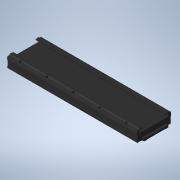
# Autodesk Inventor part: ETH2-17-L5-350-BC-M40B-C6N5L_1
Saved by Autodesk Inventor 2021 (Build 250183000, 183)
## iProperties
Created: 2025-05-01
Part Number: ETH2-17-L5-350-BC-M40B-C6N5L_1
Material: Generic
Catalog Web Link: www.cadenas.de
Description: ETH2_17_1-ETH2
Vendor: TOYO
Document SubType Name: Modeling
Designer: psAdmin
Manufacturer: TOYO
Mass: 3122.58 g
Surface Area: 3378.61 cm^2
Volume: 3122.58 cm^3
Density: 1 g/cm^3
Appearance: PSOLRGB-175-175-175
Category: PARTsolutions
Company: TOYO
Title: ETH2-17-L5-350-BC-M40B-C6N5L
Author: Cadenas PARTsolutions
Comments: ETH2
PSOL_IDENT_0: {$CADENAS_DATA/23d-libs/toyo/eth2_series/eth2_17/parts/eth2_17_body1.prj},242 {VTYP=3D},{NB=ETH2-17-
PSOL_IDENT_1: L5-350-BC-M40B-C6N5L_1},{LINA=ETH2-17-L5-350-BC-M40B-C6N5L},{NN=ETH2_17_1},{DATE=15.08.2024 07:04:56
PSOL_IDENT_2: },{GEOMDATE=05.08.2024 03:26:00},{VERSION=},{LINEID=10},{WBVAR=BSL,STROKE,MP,MB,BRAKE,HS,LS,OML,SD},
PSOL_IDENT_3: {WBNUMERIC=STROKE}  {NB=ETH2-17-L5-350-BC-M40B-C6N5L_1},{LINA=ETH2-17-L5-350-BC-M40B-C6N5L},{KT=DUMM
PSOL_IDENT_4: Y},{CNSORDERNO=ETH2-17-L5-350-BC-M40B-C6N5L},{MODEL=ETH2-17},{BSL=5},{BSL1=5},{STROKE=350},{MP=BC},{
PSOL_IDENT_5: MB=M},{POWEWR=40：400W},{BRAKE=B},{HS=C},{LS=6},{LS1='3','3:1 Pc','4','4:2 Pc','6','6:3 Pc','7','7:4
PSOL_IDENT_6: Pc','8','8:5 Pc','9','9:6 Pc','5','5:No Sensor'},{OML=N5},{SD=L},{L=615},{A=69},{A1=69},{M=4},{N=10}
PSOL_IDENT_7: ,{KG=9.42},{HLS=C6},{LSLIDER=1},{RSLIDRE=0},{MBCODE=M40B}
NB: ETH2-17-L5-350-BC-M40B-C6N5L_1
NN: ETH2_17_1
NT: ETH2
NBSYN: $CNSORDERNO._1
LINA: ETH2-17-L5-350-BC-M40B-C6N5L
CATALOG: TOYO
MODEL: ETH2-17
BSL: 5:5mm
STROKE: 350
MP: BC:Motor Exposed
MB: M:Mitsubishi
POWEWR: 40：400W
BRAKE: B:With brake
HS: C:Motor Side
LS: 6:3 Pc
OML: N5:NPN+5 meter cable
SD: L: Left side of slide
SUPPLIER: TOYO
ARTICLENO: ETH2-17-L5-350-BC-M40B-C6N5L_1
BOMINFO: ETH2-17-L5-350-BC-M40B-C6N5L
CREATOR: CADENAS GmbH
Autodesk Inventor part; units mm, degrees
sketch "__4" plane through (0, 0, 0) normal (1, 0, 0) x (0, 1, 0)
  line L0 (43, 79) -> (41.05, 79)
  arc A0 (41.05, 79) -> (40.75, 78.7) centre (41.05, 78.7) ccw
  line L1 (40.75, 78.7) -> (40.75, 77.8)
  arc A1 (40.75, 77.8) -> (41.05, 77.5) centre (41.05, 77.8) ccw
  line L2 (41.05, 77.5) -> (41.55, 77.5)
  arc A2 (41.85, 77.2) -> (41.55, 77.5) centre (41.55, 77.2) ccw
  line L3 (41.85, 77.2) -> (41.85, 75.1743)
  arc A3 (41.7621, 74.9621) -> (41.85, 75.1743) centre (41.55, 75.1743) ccw
  line L4 (41.7621, 74.9621) -> (40.6879, 73.8879)
  arc A4 (40.4757, 73.8) -> (40.6879, 73.8879) centre (40.4757, 74.1) ccw
  line L5 (40.4757, 73.8) -> (37.5243, 73.8)
  arc A5 (37.3121, 73.8879) -> (37.5243, 73.8) centre (37.5243, 74.1) ccw
  line L6 (37.3121, 73.8879) -> (36.2379, 74.9621)
  arc A6 (36.15, 75.1743) -> (36.2379, 74.9621) centre (36.45, 75.1743) ccw
  line L7 (36.15, 75.1743) -> (36.15, 77.2)
  arc A7 (36.45, 77.5) -> (36.15, 77.2) centre (36.45, 77.2) ccw
  line L8 (36.45, 77.5) -> (36.95, 77.5)
  arc A8 (36.95, 77.5) -> (37.25, 77.8) centre (36.95, 77.8) ccw
  line L9 (37.25, 77.8) -> (37.25, 78.7)
  arc A9 (37.25, 78.7) -> (36.95, 79) centre (36.95, 78.7) ccw
  line L10 (36.95, 79) -> (35, 79)
  arc A10 (35, 79) -> (34, 78) centre (35, 78) ccw
  line L11 (34, 78) -> (34, 75.8)
  arc A11 (33.5, 75.3) -> (34, 75.8) centre (33.5, 75.8) ccw
  line L12 (33.5, 75.3) -> (10.8243, 75.3)
  arc A12 (10.6121, 75.3879) -> (10.8243, 75.3) centre (10.8243, 75.6) ccw
  line L13 (10.6121, 75.3879) -> (10.0879, 75.9121)
  arc A13 (10.0879, 75.9121) -> (9.8757, 76) centre (9.8757, 75.7) ccw
  line L14 (9.8757, 76) -> (0.6243, 76)
  arc A14 (0.6243, 76) -> (0.4121, 75.9121) centre (0.6243, 75.7) ccw
  line L15 (0.4121, 75.9121) -> (0, 75.5)
  line L16 (0, 75.5) -> (0, 39.5)
  line L17 (0, 39.5) -> (0.9121, 38.5879)
  arc A15 (1, 38.3757) -> (0.9121, 38.5879) centre (0.7, 38.3757) ccw
  line L18 (1, 38.3757) -> (1, -38.3757)
  arc A16 (0.9121, -38.5879) -> (1, -38.3757) centre (0.7, -38.3757) ccw
  line L19 (0.9121, -38.5879) -> (0, -39.5)
  line L20 (0, -39.5) -> (0, -75.5)
  line L21 (0, -75.5) -> (0.5, -76)
  line L22 (0.5, -76) -> (10, -76)
  line L23 (10, -76) -> (10.6121, -75.3879)
  arc A17 (10.8243, -75.3) -> (10.6121, -75.3879) centre (10.8243, -75.6) ccw
  line L24 (10.8243, -75.3) -> (26.1757, -75.3)
  arc A18 (26.3879, -75.3879) -> (26.1757, -75.3) centre (26.1757, -75.6) ccw
  line L25 (26.3879, -75.3879) -> (28, -77)
  line L26 (28, -77) -> (45, -77)
  line L27 (45, -77) -> (46.9121, -75.0879)
  arc A19 (46.9121, -75.0879) -> (47, -74.8757) centre (46.7, -74.8757) ccw
  line L28 (47, -74.8757) -> (47, -69.3743)
  arc A20 (47.0879, -69.1621) -> (47, -69.3743) centre (47.3, -69.3743) ccw
  line L29 (47.0879, -69.1621) -> (51.4121, -64.8379)
  arc A21 (51.4121, -64.8379) -> (51.5, -64.6257) centre (51.2, -64.6257) ccw
  line L30 (51.5, -64.6257) -> (51.5, -61.9243)
  arc A22 (51.5, -61.9243) -> (51.4121, -61.7121) centre (51.2, -61.9243) ccw
  line L31 (51.4121, -61.7121) -> (51.2879, -61.5879)
  arc A23 (51.2, -61.3757) -> (51.2879, -61.5879) centre (51.5, -61.3757) ccw
  line L32 (51.2, -61.3757) -> (51.2, -56.8)
  arc A24 (51.2, -56.8) -> (50.9, -56.5) centre (50.9, -56.8) ccw
  line L33 (50.9, -56.5) -> (50.259, -56.5)
  arc A25 (49.141, -56.5) -> (50.259, -56.5) centre (49.7, -56) ccw
  line L34 (49.141, -56.5) -> (48.5, -56.5)
  arc A26 (48.2, -56.2) -> (48.5, -56.5) centre (48.5, -56.2) ccw
  line L35 (48.2, -56.2) -> (48.2, -52.8)
  arc A27 (48.5, -52.5) -> (48.2, -52.8) centre (48.5, -52.8) ccw
  line L36 (48.5, -52.5) -> (49.141, -52.5)
  arc A28 (50.259, -52.5) -> (49.141, -52.5) centre (49.7, -53) ccw
  line L37 (50.259, -52.5) -> (50.9, -52.5)
  arc A29 (50.9, -52.5) -> (51.2, -52.2) centre (50.9, -52.2) ccw
  line L38 (51.2, -52.2) -> (51.2, -51.5)
  arc A30 (51.2, -51.5) -> (50.7, -51) centre (50.7, -51.5) ccw
  line L39 (50.7, -51) -> (47, -51)
  arc A31 (47, -51) -> (45.5, -52.5) centre (47, -52.5) ccw
  line L40 (45.5, -52.5) -> (45.5, -61.3762)
  arc A32 (45.5, -61.3762) -> (45.673, -61.648) centre (45.8, -61.3762) ccw
  line L41 (45.673, -61.648) -> (45.708, -61.664)
  arc A33 (45.708, -61.664) -> (46.084, -61.559) centre (45.8347, -61.3921) ccw
  arc A34 (46.269, -63.673) -> (46.084, -61.559) centre (47.4997, -62.5002) ccw
  arc A35 (46.269, -63.673) -> (45.8797, -63.6342) centre (46.0518, -63.8799) ccw
  line L42 (45.8797, -63.6342) -> (43.4739, -65.3191)
  arc A36 (42.9002, -65.5) -> (43.4739, -65.3191) centre (42.9002, -64.5) ccw
  line L43 (42.9002, -65.5) -> (32.748, -65.5)
  line L44 (32.748, -65.5) -> (32.748, 65.5)
  line L45 (32.748, 65.5) -> (42.9002, 65.5)
  arc A37 (43.4739, 65.3191) -> (42.9002, 65.5) centre (42.9002, 64.5) ccw
  line L46 (43.4739, 65.3191) -> (45.8797, 63.6342)
  arc A38 (45.8797, 63.6342) -> (46.269, 63.673) centre (46.0518, 63.8799) ccw
  arc A39 (46.084, 61.559) -> (46.269, 63.673) centre (47.4997, 62.5002) ccw
  arc A40 (46.084, 61.559) -> (45.708, 61.664) centre (45.8347, 61.3921) ccw
  line L47 (45.708, 61.664) -> (45.673, 61.648)
  arc A41 (45.673, 61.648) -> (45.5, 61.3762) centre (45.8, 61.3762) ccw
  line L48 (45.5, 61.3762) -> (45.5, 52.5)
  arc A42 (45.5, 52.5) -> (47, 51) centre (47, 52.5) ccw
  line L49 (47, 51) -> (50.7, 51)
  arc A43 (50.7, 51) -> (51.2, 51.5) centre (50.7, 51.5) ccw
  line L50 (51.2, 51.5) -> (51.2, 52.2)
  arc A44 (51.2, 52.2) -> (50.9, 52.5) centre (50.9, 52.2) ccw
  line L51 (50.9, 52.5) -> (50.259, 52.5)
  arc A45 (49.141, 52.5) -> (50.259, 52.5) centre (49.7, 53) ccw
  line L52 (49.141, 52.5) -> (48.5, 52.5)
  arc A46 (48.2, 52.8) -> (48.5, 52.5) centre (48.5, 52.8) ccw
  line L53 (48.2, 52.8) -> (48.2, 56.2)
  arc A47 (48.5, 56.5) -> (48.2, 56.2) centre (48.5, 56.2) ccw
  line L54 (48.5, 56.5) -> (49.141, 56.5)
  arc A48 (50.259, 56.5) -> (49.141, 56.5) centre (49.7, 56) ccw
  line L55 (50.259, 56.5) -> (50.9, 56.5)
  arc A49 (50.9, 56.5) -> (51.2, 56.8) centre (50.9, 56.8) ccw
  line L56 (51.2, 56.8) -> (51.2, 61.3757)
  arc A50 (51.2879, 61.5879) -> (51.2, 61.3757) centre (51.5, 61.3757) ccw
  line L57 (51.2879, 61.5879) -> (51.4121, 61.7121)
  arc A51 (51.4121, 61.7121) -> (51.5, 61.9243) centre (51.2, 61.9243) ccw
  line L58 (51.5, 61.9243) -> (51.5, 64.6257)
  arc A52 (51.5, 64.6257) -> (51.4121, 64.8379) centre (51.2, 64.6257) ccw
  line L59 (51.4121, 64.8379) -> (47.0879, 69.1621)
  arc A53 (47, 69.3743) -> (47.0879, 69.1621) centre (47.3, 69.3743) ccw
  line L60 (47, 69.3743) -> (47, 74.8757)
  arc A54 (47, 74.8757) -> (46.9121, 75.0879) centre (46.7, 74.8757) ccw
  line L61 (46.9121, 75.0879) -> (46.0879, 75.9121)
  arc A55 (46.0879, 75.9121) -> (45.8757, 76) centre (45.8757, 75.7) ccw
  line L62 (45.8757, 76) -> (44.5, 76)
  arc A56 (44, 76.5) -> (44.5, 76) centre (44.5, 76.5) ccw
  line L63 (44, 76.5) -> (44, 78)
  arc A57 (44, 78) -> (43, 79) centre (43, 78) ccw
  constraints: 128 end point, 116 point on circle, 58 centre point
extrude "Extrusion1" add sketch "__4" along normal blind 596
sketch "__1" plane through (0, 0, 0) normal (0, 1, 0) x (-1, 0, 0)
  line L0 (-586, 90) -> (-606, 90)
  line L1 (-606, 90) -> (-606, -90)
  line L2 (-606, -90) -> (-586, -90)
  line L3 (-586, -90) -> (-586, -60.5)
  arc A0 (-586, -60.5) -> (-592, -54.5) centre (-592, -60.5) ccw
  line L4 (-592, -54.5) -> (-596, -54.5)
  line L5 (-596, -54.5) -> (-596, 54.5)
  line L6 (-596, 54.5) -> (-592, 54.5)
  arc A1 (-592, 54.5) -> (-586, 60.5) centre (-592, 60.5) ccw
  line L7 (-586, 60.5) -> (-586, 90)
  constraints: 16 end point, 4 point on circle, 2 centre point
extrude "Extrusion2" cut sketch "__1" along normal blind 51.5
sketch "__3" plane through (596, 0, 0) normal (1, 0, 0) x (0, 0, -1)
  line L0 (-90, 70) -> (-90, 0)
  line L1 (-90, 0) -> (-60.5, 0)
  line L2 (-60.5, 0) -> (-60.5, 12.8)
  line L3 (-60.5, 12.8) -> (-58.4243, 12.8)
  arc A0 (-58.2121, 12.7121) -> (-58.4243, 12.8) centre (-58.4243, 12.5) ccw
  line L4 (-58.2121, 12.7121) -> (-56.0879, 10.5879)
  arc A1 (-56.0879, 10.5879) -> (-55.8757, 10.5) centre (-55.8757, 10.8) ccw
  line L5 (-55.8757, 10.5) -> (-55.6243, 10.5)
  arc A2 (-55.6243, 10.5) -> (-55.4121, 10.5879) centre (-55.6243, 10.8) ccw
  line L6 (-55.4121, 10.5879) -> (-55, 11)
  line L7 (-55, 11) -> (-39, 11)
  line L8 (-39, 11) -> (-37.5879, 9.5879)
  arc A3 (-37.5879, 9.5879) -> (-37.3757, 9.5) centre (-37.3757, 9.8) ccw
  line L9 (-37.3757, 9.5) -> (-30.1243, 9.5)
  arc A4 (-30.1243, 9.5) -> (-29.9121, 9.5879) centre (-30.1243, 9.8) ccw
  line L10 (-29.9121, 9.5879) -> (-29.5, 10)
  line L11 (-29.5, 10) -> (-17.5, 10)
  line L12 (-17.5, 10) -> (-17.0879, 9.5879)
  arc A5 (-17.0879, 9.5879) -> (-16.8757, 9.5) centre (-16.8757, 9.8) ccw
  line L13 (-16.8757, 9.5) -> (16.8757, 9.5)
  arc A6 (16.8757, 9.5) -> (17.0879, 9.5879) centre (16.8757, 9.8) ccw
  line L14 (17.0879, 9.5879) -> (17.5, 10)
  line L15 (17.5, 10) -> (27.634, 10)
  arc A7 (27.634, 10) -> (29, 11.366) centre (28.5001, 10.4999) ccw
  line L16 (29, 11.366) -> (29, 12)
  line L17 (29, 12) -> (30.8757, 12)
  arc A8 (31.0879, 11.9121) -> (30.8757, 12) centre (30.8757, 11.7) ccw
  line L18 (31.0879, 11.9121) -> (32.5121, 10.4879)
  arc A9 (32.5121, 10.4879) -> (32.7243, 10.4) centre (32.7243, 10.7) ccw
  line L19 (32.7243, 10.4) -> (38.2757, 10.4)
  arc A10 (38.2757, 10.4) -> (38.4879, 10.4879) centre (38.2757, 10.7) ccw
  line L20 (38.4879, 10.4879) -> (39, 11)
  line L21 (39, 11) -> (53.134, 11)
  arc A11 (53.134, 11) -> (54.5, 10.634) centre (54, 11.5) ccw
  arc A12 (54.5, 10.634) -> (54.866, 11) centre (54, 11.5) ccw
  line L22 (54.866, 11) -> (60.5, 11)
  line L23 (60.5, 11) -> (60.5, 0)
  line L24 (60.5, 0) -> (90, 0)
  line L25 (90, 0) -> (90, 70)
  line L26 (90, 70) -> (-90, 70)
  constraints: 54 end point, 26 point on circle, 13 centre point
extrude "Extrusion3" cut sketch "__3" against normal blind 10
sketch "__5" plane through (0, 0, 70) normal (0, 0, 1) x (1, 0, 0)
  line L0 (51, 51.5) -> (51, 0)
  line L1 (51, 0) -> (48, 0)
  line L2 (48, 0) -> (48.5415, 0.5415)
  line L3 (48.5415, 0.5415) -> (48.5415, 45.5)
  line L4 (48.5415, 45.5) -> (46.25, 45.5)
  line L5 (46.25, 45.5) -> (46.25, 51.5)
  line L6 (46.25, 51.5) -> (51, 51.5)
  line L7 (51, 51.5) -> (51, 0)
  constraints: 16 end point
revolve "Revolution1" cut sketch "__5" angle 360 about axis through (51, 51.5, 70) along (0, 1, 0)
thread "Thread1" size "M6x1" class "6H" standard "ISO Metric profile" full length
pattern_linear "Rectangular Pattern1" count 5 spacing 120 along (1, 0, 0) count 2 spacing 140 along (0, 0, -1) of "Revolution1"
sketch "Sketch5" plane through (0, 0, -75.5) normal (0, -1, 0) x (1, 0, 0)
  point P0 (8, 31)
hole "Hole1" at (8, 0, -44.5) direction (0, 1, 0) diameter 5 depth 7
pattern_linear "Rectangular Pattern2" count 2 spacing 12 along (1, 0, 0) count 2 spacing 89 along (0, 0, 1) of "Hole1"
sketch "__16" plane through (0, 0, 0) normal (0, 1, 0) x (-1, 0, 0)
  circle A0 centre (-79, 0) radius 2.1
  constraints: 1 centre point
extrude "Extrusion4" cut sketch "__16" along normal blind 7
sketch "Pattern_3___16_0" plane through (0, 0, -23.5) normal (0, 1, 0) x (1, 0, 0)
  circle A0 centre (79, 0) radius 2.1
  constraints: 1 centre point
extrude "Extrusion5" cut sketch "Pattern_3___16_0" along normal blind 7
sketch "Pattern_3___16_1" plane through (0, 0, 23.5) normal (0, 1, 0) x (1, 0, 0)
  circle A0 centre (79, 0) radius 2.1
  constraints: 1 centre point
extrude "Extrusion6" cut sketch "Pattern_3___16_1" along normal blind 7
sketch "Pattern_3___16_2" plane through (495.5, 0, 0) normal (0, 1, 0) x (1, 0, 0)
  circle A0 centre (79, 0) radius 2.1
  constraints: 1 centre point
extrude "Extrusion7" cut sketch "Pattern_3___16_2" along normal blind 7
sketch "Pattern_3___16_3" plane through (495.5, 0, -23.5) normal (0, 1, 0) x (1, 0, 0)
  circle A0 centre (79, 0) radius 2.1
  constraints: 1 centre point
extrude "Extrusion8" cut sketch "Pattern_3___16_3" along normal blind 7
sketch "Pattern_3___16_4" plane through (495.5, 0, 23.5) normal (0, 1, 0) x (1, 0, 0)
  circle A0 centre (79, 0) radius 2.1
  constraints: 1 centre point
extrude "Extrusion9" cut sketch "Pattern_3___16_4" along normal blind 7
sketch "Sketch12" plane through (0, 0, -75.5) normal (0, -1, 0) x (1, 0, 0)
  point P0 (51, 28.5)
hole "Hole2" at (51, 0, -47) direction (0, 1, 0) diameter 3.2 depth 7
pattern_linear "Rectangular Pattern3" count 9 spacing 60 along (1, 0, 0) count 2 spacing 94 along (0, 0, 1) of "Hole2"
ref_plane "BODYY_XY" through (596.5, 1.68, 0) normal (-1, 0, 0) x (0, 0, -1)
ref_plane "BODYY_YZ" through (596.5, 1.68, 0) normal (0, 0, -1) x (0, -1, 0)
ref_plane "BODYY_ZX" through (596.5, 1.68, 0) normal (0, -1, 0) x (-1, 0, 0)
ref_plane "BODYZ_XY" through (0, 1.5, 0) normal (1, 0, 0) x (0, 0, -1)
ref_plane "BODYZ_YZ" through (0, 1.5, 0) normal (0, 0, -1) x (0, 1, 0)
ref_plane "BODYZ_ZX" through (0, 1.5, 0) normal (0, 1, 0) x (1, 0, 0)
ref_plane "DAOGUI_XY" through (0, 51.5, 0) normal (-1, 0, 0) x (0, 0, -1)
ref_plane "DAOGUI_YZ" through (0, 51.5, 0) normal (0, 0, -1) x (0, -1, 0)
ref_plane "DAOGUI_ZX" through (0, 51.5, 0) normal (0, -1, 0) x (-1, 0, 0)
ref_plane "DUMMY_XY" through (0, 0, 0) normal (-1, 0, 0) x (0, 0, -1)
ref_plane "DUMMY_YZ" through (0, 0, 0) normal (0, 0, -1) x (0, -1, 0)
ref_plane "DUMMY_ZX" through (0, 0, 0) normal (0, -1, 0) x (-1, 0, 0)
ref_plane "HUATAI_XY" through (126, 35, 0) normal (-1, 0, 0) x (0, 0, -1)
ref_plane "HUATAI_YZ" through (126, 35, 0) normal (0, 0, -1) x (0, -1, 0)
ref_plane "HUATAI_ZX" through (126, 35, 0) normal (0, -1, 0) x (-1, 0, 0)
ref_plane "SENOR_L_XY" through (143.5, 39, 79) normal (-1, 0, 0) x (0, 0, -1)
ref_plane "SENOR_L_YZ" through (143.5, 39, 79) normal (0, 0, -1) x (0, -1, 0)
ref_plane "SENOR_L_ZX" through (143.5, 39, 79) normal (0, -1, 0) x (-1, 0, 0)
ref_plane "SENOR_R_XY" through (143.5, 39, -79) normal (1, 0, 0) x (0, 0, -1)
ref_plane "SENOR_R_YZ" through (143.5, 39, -79) normal (0, 0, -1) x (0, 1, 0)
ref_plane "SENOR_R_ZX" through (143.5, 39, -79) normal (0, 1, 0) x (1, 0, 0)
body "Solid1"
